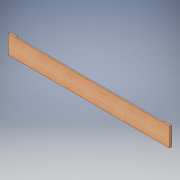
# Autodesk Inventor part: SkinnySideL
Saved by Autodesk Inventor 2016 (Build 200138000, 138)
## iProperties
Created: 2016-02-11
Part Number: SkinnySideL
Material: Wood (Birch)
Document SubType Name: Modeling
Designer: ron
Density: 0.55 g/cm^3
Appearance: Birch - Natural Polished
Mass: 1942.9 g
Surface Area: 4803.23 cm^2
Volume: 3532.55 cm^3
Author: ron
Autodesk Inventor part; units mm, degrees
ref_plane "YZ Plane" through (0, 0, 0) normal (1, 0, 0) x (0, 1, 0)
ref_plane "XZ Plane" through (0, 0, 0) normal (0, 1, 0) x (-1, 0, 0)
ref_plane "XY Plane" through (0, 0, 0) normal (0, 0, 1) x (1, 0, 0)
sketch "Sketch1" plane through (0, 0, 0) normal (1, 0, 0) x (0, 1, 0)
  line L0 (0, 0) -> (155.1, 0)
  line L1 (155.1, 0) -> (155.1, -10)
  line L2 (0, -20) -> (0, 0)
  line L3 (155.1, -10) -> (101.6, -10)
  line L4 (101.6, -10) -> (101.6, -20)
  line L5 (101.6, -20) -> (0, -20)
  dimension "d3" = 53.5
  dimension "d4" = 155.1
  dimension "d5" = 10
  dimension "d6" = 10
  dimension "d7" = 20
  dimension "d18" = 101.6
  constraints: 12 end point, 3 horizontal, 2 parallel, 1 perpendicular
  measures "d3" distance of L1.end L3.end
  measures "d4" distance between parallel lines of L1 L2
  measures "d5" distance between parallel lines of L3 L5
  measures "d6" distance between parallel lines of L0 L3
  measures "d7" vertical distance of L4.end L0.end
  measures "d18" distance of L4.end L2.start
extrude "Extrusion1" add sketch "Sketch1" along normal blind 1350.7974
sketch "Sketch3" plane through (0, 101.6, -10) normal (0, 1, 0) x (1, 0, 0)
  line L0 (1350.7974, -10) -> (1350.7974, 10) projected
  line L1 (1350.7974, 10) -> (1289.9898, 10)
  line L2 (1289.9898, 10) -> (1289.9898, 0)
  line L3 (0, 0) -> (1350.7974, 0) projected
  line L4 (0, 10) -> (0, -10) projected
  line L5 (0, 10) -> (60.8076, 10)
  line L6 (60.8076, 10) -> (60.8076, 0)
  dimension "d19" = 60.8076
  dimension "d20" = 60.8076
  constraints: 8 end point, 2 perpendicular, 2 point on line
  measures "d19" distance of L0.end L1.end
  measures "d20" distance of L4.start L5.end
extrude "Extrusion2" add sketch "Sketch3" along normal blind 53.4924 contours L3 L2 L1 L0
sketch "Sketch4" plane through (0, 101.6, -20) normal (0, 1, 0) x (1, 0, 0)
  line L0 (1350.7974, -10) -> (1350.7974, 10)
  line L1 (1350.7974, 10) -> (1289.9898, 10)
  line L2 (1289.9898, 10) -> (1289.9898, 0)
  line L3 (0, 0) -> (1350.7974, 0)
  line L4 (0, 10) -> (60.8076, 10)
  line L5 (60.8076, 10) -> (60.8076, 0)
  line L6 (0, 10) -> (0, 0)
  line L7 (0, -20) -> (0, -10) projected
  line L8 (0, 0) -> (0, -20)
  line L9 (60.8076, 0) -> (60.8076, -10)
  line L10 (0, -10) -> (1350.7974, -10) projected
  line L11 (0, -10) -> (60.8076, -10)
  line L12 (0, -10) -> (0, 0)
  dimension "d23" = 60.8076
  dimension "d24" = 60.8076
  dimension "d25" = 10
  dimension "d26" = 20
  constraints: 22 end point, 4 vertical, 3 point on line, 2 perpendicular, 1 collinear
  measures "d23" distance of L0.end L1.end
  measures "d24" distance of L4.start L4.end
  measures "d25" distance of L3.start L4.start
  measures "d26" distance of L3.start L7.start
extrude "Extrusion3" add sketch "Sketch4" along normal blind 53.4924 contours L10 L8 L3 L9
body "Solid1"
